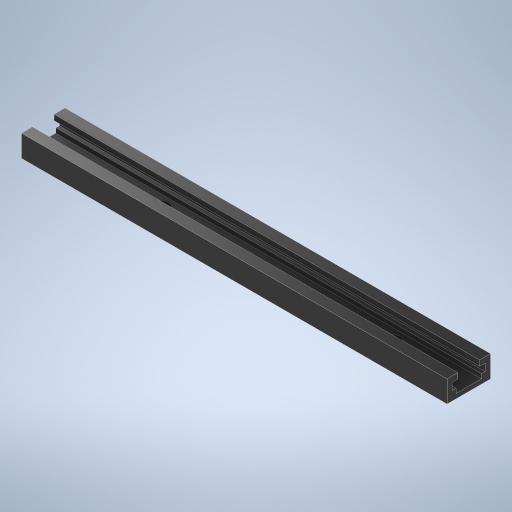
# Autodesk Inventor part: C-Channel_7.334in
Saved by Autodesk Inventor 2024 (Build 280153000, 153)
## iProperties
Created: 2023-06-15
Part Number: C-Channel_7.334in
Material: Generic
Document SubType Name: Modeling
Designer: 18179
Density: 1 g/cm^3
Appearance: Glossy - Black
Author: 18179
Autodesk Inventor part; units mm, degrees
ref_plane "YZ Plane" through (0, 0, 0) normal (1, 0, 0) x (0, 1, 0)
ref_plane "XZ Plane" through (0, 0, 0) normal (0, 1, 0) x (-1, 0, 0)
ref_plane "XY Plane" through (0, 0, 0) normal (0, 0, 1) x (1, 0, 0)
sketch "Sketch1" plane through (0, 0, 0) normal (1, 0, 0) x (0, 1, 0)
  line L0 (0, 0) -> (9.525, 0)
  line L1 (9.525, 0) -> (9.525, -19.05)
  line L2 (9.525, -19.05) -> (0, -19.05)
  line L3 (0, -19.05) -> (0, 0)
  line L4 (0, 0) -> (7.1437, 0)
  line L5 (7.1437, 0) -> (7.1437, -19.05) construction
  line L6 (0, 0) -> (3.9688, 0) construction
  line L7 (3.9688, 0) -> (3.9688, -19.231) construction
  line L8 (9.525, -9.525) -> (9.525, -2.3813) construction
  line L9 (9.525, -9.525) -> (9.525, -4.7625)
  line L10 (9.525, -4.7625) -> (7.1437, -4.7625)
  line L11 (7.1437, -4.7625) -> (7.1437, -2.3813)
  line L12 (9.525, -9.525) -> (12.141, -9.525)
  line L13 (7.1437, -2.3813) -> (3.9688, -2.3813)
  line L14 (9.525, -9.525) -> (9.525, -3.9688)
  line L15 (9.525, -3.9688) -> (0, -3.9687) construction
  line L16 (3.9688, -2.3813) -> (3.9688, -3.9687)
  line L17 (1.9844, -3.9687) -> (3.9688, -3.9687)
  line L18 (1.9844, -3.9687) -> (1.9844, -9.525)
  line L19 (9.525, -14.2875) -> (7.1437, -14.2875)
  line L20 (7.1437, -14.2875) -> (7.1437, -16.6687)
  line L21 (7.1437, -16.6687) -> (3.9688, -16.6687)
  line L22 (3.9688, -16.6687) -> (3.9688, -15.0813)
  line L23 (1.9844, -15.0813) -> (3.9688, -15.0813)
  line L24 (1.9844, -15.0813) -> (1.9844, -9.525)
  dimension "d20" = 9.525
  dimension "d21" = 19.05
  dimension "d22" = 7.1437
  dimension "d23" = 3.9688
  dimension "d24" = 7.1437
  dimension "d25" = 4.7625
  dimension "d26" = 5.5563
  constraints: 50 end point, 12 point on line, 6 perpendicular, 6 symmetric about line, 2 collinear, 2 horizontal, 2 parallel, 1 midpoint, 1 vertical
  measures "d20" distance of L1.end L2.end
  measures "d21" distance of L0.end L1.end
  measures "d22" distance of L0.start L4.end
  measures "d23" distance of L0.start L6.end
  measures "d24" distance of L8.start L8.end
  measures "d25" distance of L8.start L9.end
  measures "d26" distance of L8.start L14.end
extrude "Extrusion1" add sketch "Sketch1" along normal blind 186.2836 contours L0 L1 L10 L11 L13 L16 L17 L18 L24 L23 L22 L21 L20 L19 L2 L3
sketch "Sketch2" plane through (0, 1.9844, -3.9687) normal (0, 1, 0) x (1, 0, 0)
  line L0 (0, 11.1125) -> (0, 0) projected
  line L1 (0, 0) -> (186.2836, 0) projected
  line L2 (186.2836, 11.1125) -> (186.2836, 0) projected
  line L3 (0, 11.1125) -> (186.2836, 11.1125) projected
  line L4 (0, 5.5563) -> (50.8, 5.5563)
  line L5 (50.8, 5.5563) -> (152.4, 5.5563)
  line L6 (152.4, 5.5563) -> (50.8, 5.5563)
  line L7 (50.8, 5.5563) -> (254, 5.5563)
  circle A0 centre (50.8, 5.5563) radius 3.9687
  circle A1 centre (152.4, 5.5563) radius 3.9687
  circle A2 centre (254, 5.5563) radius 3.9687
  line L8 (93.1418, 0) -> (93.1418, 17.8436)
  circle A3 centre (-67.7164, 5.5563) radius 3.9687
  point P0 (0, -3.9687)
  dimension "d27" = 50.8
  dimension "d28" = 101.6
  dimension "d29" = 101.6
  dimension "d30" = 203.2
  dimension "d31" = 7.9375
  dimension "d32" = 7.9375
  dimension "d33" = 7.9375
  constraints: 10 end point, 4 centre point, 3 coincident, 2 midpoint, 2 point on line, 1 collinear, 1 horizontal, 1 symmetric about line, 1 vertical, 1 other
  measures "d27" distance of L4.start L4.end
  measures "d28" distance of L4.end L5.end
  measures "d29" distance of L5.end L4.end
  measures "d30" distance of L4.end L7.end
  measures "d31" diameter of A0
  measures "d32" diameter of A1
  measures "d33" diameter of A2
extrude "Extrusion2" cut sketch "Sketch2" against normal through all contours A2 | A0 L5 L4 | L4 L5 A0 | A1 L7 L5 | L5 L7 A1 | A3
body "Solid1"
